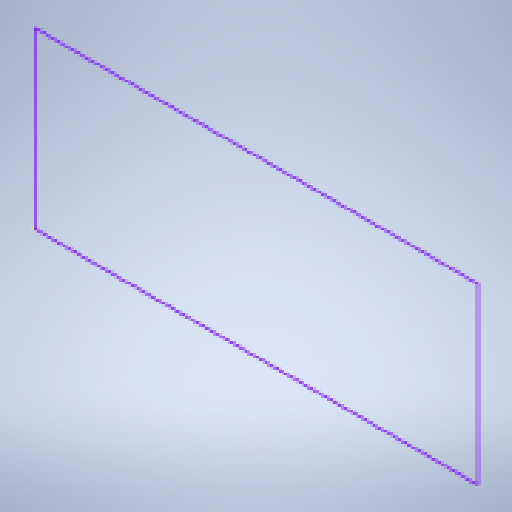
# Autodesk Inventor part: support pile
Saved by Autodesk Inventor 2024 (Build 280153000, 153)
## iProperties
Created: 2024-03-05
Part Number: support pile
Material: Générique
Document SubType Name: Modeling
Designer: phaly
Density: 1 g/cm^3
Appearance: Par défaut
Author: phaly
Autodesk Inventor part; units mm, degrees
ref_plane "YZ Plane" through (0, 0, 0) normal (1, 0, 0) x (0, 1, 0)
ref_plane "XZ Plane" through (0, 0, 0) normal (0, 1, 0) x (-1, 0, 0)
ref_plane "XY Plane" through (0, 0, 0) normal (0, 0, 1) x (1, 0, 0)
sketch "Esquisse1" plane through (0, 0, 0) normal (0, 0, 1) x (1, 0, 0)
  line L0 (0, 21) -> (40, 21)
  line L1 (40, 21) -> (40, 0)
  line L2 (40, 0) -> (0, 0)
  line L3 (0, 0) -> (0, 21)
  line L4 (-8, 0) -> (48, 0) projected
  line L5 (0, -4.2) -> (0, 25.2) projected
  point P0 (0, 0)
  dimension "d0" = 40
  dimension "d1" = 21
  constraints: 8 end point, 2 collinear, 2 parallel, 1 horizontal, 1 perpendicular
  measures "d0" distance of L0.start L0.end
  measures "d1" distance of L0.end L1.end
extrude "Extrusion1" add sketch "Esquisse1" along normal mid plane 73
sketch "Esquisse2" plane through (0, 0, 36.5) normal (0, 0, 1) x (1, 0, 0)
  circle A0 centre (10, 10.5) radius 7
  circle A1 centre (30, 10.5) radius 7
  line L0 (40, 21) -> (0, 21) projected
  line L1 (0, 21) -> (0, 0) projected
  line L2 (40, 0) -> (40, 21) projected
  line L3 (0, 0) -> (40, 0) projected
  dimension "d4" = 14
  dimension "d5" = 14
  dimension "d11" = 10.5
  dimension "d20" = 10.5
  dimension "d21" = 20
  constraints: 2 centre point
  measures "d4" diameter of A0
  measures "d5" diameter of A1
  measures "d11" distance from line of L3 A1.centre
  measures "d20" distance from line of L3 A0.centre
  measures "d21" distance of A1.centre A0.centre
extrude "Extrusion2" cut sketch "Esquisse2" against normal through all contours A0 | A1
sketch "Esquisse3" plane through (0, 21, 36.5) normal (0, 1, 0) x (1, 0, 0)
  line L0 (2, 71) -> (38, 71)
  line L1 (38, 71) -> (38, 2)
  line L2 (38, 2) -> (2, 2)
  line L3 (2, 2) -> (2, 71)
  line L4 (0, 73) -> (40, 73) projected
  line L5 (40, 0) -> (0, 0) projected
  line L6 (40, 73) -> (40, 0) projected
  line L7 (0, 73) -> (0, 0) projected
  point P0 (0, 36.5)
  dimension "d14" = 2
  dimension "d15" = 2
  dimension "d16" = 2
  dimension "d17" = 2
  constraints: 8 end point, 2 parallel, 1 horizontal, 1 perpendicular
  measures "d14" distance between parallel lines of L4 L0
  measures "d15" distance between parallel lines of L5 L2
  measures "d16" distance between parallel lines of L6 L1
  measures "d17" distance between parallel lines of L7 L3
extrude "Extrusion3" cut sketch "Esquisse3" against normal blind 14 contours L0 L1 L2 L3
equation "\"d5\" = d4"
equation "\"d11\" = d20"
equation "\"d15\" = d14"
equation "\"d16\" = d15"
equation "\"d17\" = d16"
